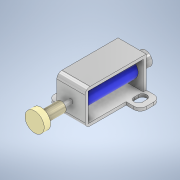
# Autodesk Inventor part: Solenoid
Saved by Autodesk Inventor 2021 (Build 250183000, 183)
## iProperties
Created: 2021-02-15
Part Number: Solenoid
Material: Generic
Document SubType Name: Modeling
Designer: Ryan
Density: 1 g/cm^3
Appearance: Default
Author: Ryan
Autodesk Inventor part; units mm, degrees
ref_plane "YZ Plane" through (0, 0, 0) normal (1, 0, 0) x (0, 1, 0)
ref_plane "XZ Plane" through (0, 0, 0) normal (0, 1, 0) x (-1, 0, 0)
sketch "Sketch1" plane through (0, 0, 0) normal (0, 1, 0) x (-1, 0, 0)
  line L0 (7, 15.2) -> (-7, 15.2)
  line L1 (-7, 15.2) -> (-7, -15.2)
  line L2 (-7, -15.2) -> (7, -15.2)
  line L3 (7, -15.2) -> (7, 15.2)
  point P0 (0, 0)
  dimension "d0" = 30.4
  dimension "d1" = 14
  dimension "d2" = 7
  dimension "d3" = 15.2
  constraints: 8 end point, 2 parallel, 1 horizontal, 1 perpendicular
  measures "d0" distance of L2.end L0.start
  measures "d1" distance of L0.start L0.end
  measures "d2" distance from line of point (0, 0) L3
  measures "d3" distance from line of point (0, 0) L0
extrude "Extrusion1" add sketch "Sketch1" along normal blind 17
fillet "Fillet1" radius 2.54 2 edges at (0, 17, 15.2) (0, 0, 15.2)
sketch "Sketch2" plane through (7, 0, -15.2) normal (1, 0, 0) x (0, 0, -1)
  line L0 (-1.5, 15.5) -> (-28.9, 15.5)
  line L1 (-28.9, 15.5) -> (-28.9, 1.5)
  line L2 (-28.9, 1.5) -> (-1.5, 1.5)
  line L3 (-1.5, 1.5) -> (-1.5, 15.5)
  line L4 (-28.9, 8.5) -> (-30.4, 8.5) construction
  line L5 (-30.4, 2.54) -> (-30.4, 14.46) projected
  line L6 (-1.5, 9.1916) -> (0, 9.1916) construction
  line L7 (0, 0) -> (0, 17) projected
  line L8 (-13.3503, 1.5) -> (-13.3503, 0) construction
  line L9 (-15.2, 15.5) -> (-15.2, 17) construction
  line L10 (0, 17) -> (-27.86, 17) projected
  line L11 (-27.86, 0) -> (0, 0) projected
  point P0 (-15.2, 0)
  dimension "d7" = 1.5
  constraints: 16 end point, 5 point on line, 3 equal length, 3 midpoint, 3 parallel, 2 horizontal, 2 vertical, 1 perpendicular
  measures "d7" distance between parallel lines of L11 L2
extrude "Extrusion2" cut sketch "Sketch2" against normal blind 17
ref_plane "Work Plane1" through (0, 8.5, 0) normal (0, 1, 0) x (1, 0, 0)
sketch "Sketch4" plane through (0, 17, 0) normal (0, 1, 0) x (1, 0, 0)
  line L0 (7, 15.2) -> (-7, 15.2) projected
  line L1 (0, 15.2) -> (3.45, 15.2)
  line L2 (3.45, 15.2) -> (3.45, 21.8)
  line L3 (3.45, 21.8) -> (0, 21.8)
  line L4 (0, 21.8) -> (0, 15.2)
  line L5 (-7, -15.2) -> (7, -15.2) projected
  line L6 (0, 15.2) -> (4.5, 15.2)
  line L7 (4.5, 15.2) -> (4.5, -15.2)
  line L8 (4.5, -15.2) -> (0, -15.2)
  line L9 (0, -15.2) -> (0, 15.2)
  line L10 (1, -15.2) -> (0, -15.2)
  line L11 (0, -15.2) -> (0, -20.1)
  line L12 (0, -20.1) -> (1, -20.1)
  line L13 (1, -20.1) -> (1, -15.2)
  line L14 (0, -20.1) -> (2.5, -20.1)
  line L15 (2.5, -20.1) -> (2.5, -30.1)
  line L16 (2.5, -30.1) -> (0, -30.1)
  line L17 (0, -30.1) -> (0, -20.1)
  point P0 (0, 0)
  dimension "d10" = 3.45
  dimension "d11" = 51.9
  dimension "d12" = 10
  dimension "d14" = 4.9
  dimension "d15" = 2.5
  dimension "d16" = 1
  dimension "d17" = 4.5
  constraints: 32 end point, 8 parallel, 4 horizontal, 4 perpendicular, 3 point on line, 1 midpoint
  measures "d10" distance of L2.end L3.end
  measures "d11" distance between parallel lines of L16 L3
  measures "d12" distance of L14.end L15.end
  measures "d14" distance of L12.end L10.start
  measures "d15" distance of L15.end L16.end
  measures "d16" distance between parallel lines of L11 L13
  measures "d17" distance between parallel lines of L9 L7
sketch "Sketch5" plane through (0, 8.5, 0) normal (0, 1, 0) x (1, 0, 0)
  line L0 (0, 15.2) -> (3.45, 15.2)
  line L1 (3.45, 15.2) -> (3.45, 21.8)
  line L2 (3.45, 21.8) -> (0, 21.8)
  line L3 (0, 21.8) -> (0, 15.2)
  line L4 (0, 15.2) -> (4.5, 15.2)
  line L5 (4.5, 15.2) -> (4.5, -15.2)
  line L6 (4.5, -15.2) -> (0, -15.2)
  line L7 (0, -15.2) -> (0, 15.2)
  line L8 (1, -15.2) -> (0, -15.2)
  line L9 (0, -15.2) -> (0, -20.1)
  line L10 (0, -20.1) -> (1, -20.1)
  line L11 (1, -20.1) -> (1, -15.2)
  line L12 (0, -20.1) -> (2.5, -20.1)
  line L13 (2.5, -20.1) -> (2.5, -30.1)
  line L14 (2.5, -30.1) -> (0, -30.1)
  line L15 (0, -30.1) -> (0, -20.1)
  point P0 (0, 0)
  dimension "d18" = 3.45
  dimension "d19" = 51.9
  dimension "d20" = 10
  dimension "d21" = 4.9
  dimension "d22" = 2.5
  dimension "d23" = 1
  dimension "d24" = 4.5
  constraints: 32 end point, 8 parallel, 4 horizontal, 4 perpendicular, 2 point on line
  measures "d18" distance of L1.end L2.end
  measures "d19" distance between parallel lines of L14 L2
  measures "d20" distance of L12.end L13.end
  measures "d21" distance of L10.end L8.start
  measures "d22" distance of L13.end L14.end
  measures "d23" distance between parallel lines of L9 L11
  measures "d24" distance between parallel lines of L7 L5
revolve "Revolution1" add sketch "Sketch5" angle 360 about axis through (0, 8.5, 30.1) along (0, 0, -1)
sketch "Sketch6" plane through (0, 0, 0) normal (0, 1, 0) x (-1, 0, 0)
  line L0 (-7, -15.2) -> (7, -15.2) projected
  line L1 (-7, 12.66) -> (7, 12.66) projected
  line L2 (7, 12.66) -> (10.825, 12.66)
  line L3 (14, 9.485) -> (14, 5.835)
  line L4 (10.825, 2.66) -> (7, 2.66)
  line L5 (7, 2.66) -> (7, 12.66)
  line L6 (11.25, 6.66) -> (7, 6.66)
  line L7 (7, 6.66) -> (7, 8.66)
  line L8 (7, 8.66) -> (11.25, 8.66)
  line L9 (11.25, 8.66) -> (11.25, 6.66)
  line L10 (7, -15.2) -> (7, 12.66) projected
  line L11 (7, 7.66) -> (14, 7.66) construction
  circle A0 centre (9.125, 6.66) radius 2.125
  circle A1 centre (9.125, 8.66) radius 2.125
  arc A2 (10.825, 2.66) -> (14, 5.835) centre (10.825, 5.835) ccw
  arc A3 (14, 9.485) -> (10.825, 12.66) centre (10.825, 9.485) ccw
  line L12 (-1, 15.2) -> (1, 15.2) projected
  line L13 (7, -15.2) -> (7, 12.66) projected
  line L14 (7, 12.66) -> (7, -15.2)
  line L15 (7, -1.27) -> (-7, -1.27) construction
  line L16 (-7, -13.7) -> (-7, 13.7) projected
  line L17 (0, -1.27) -> (0, -15.2) construction
  line L18 (7, -15.2) -> (10.825, -15.2) construction
  line L19 (14, -12.025) -> (14, -8.375) construction
  line L20 (10.825, -5.2) -> (7, -5.2) construction
  line L21 (7, -5.2) -> (7, -15.2) construction
  line L22 (11.25, -9.2) -> (7, -9.2) construction
  line L23 (7, -9.2) -> (7, -11.2) construction
  line L24 (7, -11.2) -> (11.25, -11.2) construction
  line L25 (11.25, -11.2) -> (11.25, -9.2) construction
  line L26 (7, -10.2) -> (14, -10.2) construction
  circle A4 centre (9.125, -9.2) radius 2.125 construction
  circle A5 centre (9.125, -11.2) radius 2.125 construction
  arc A6 (14, -8.375) -> (10.825, -5.2) centre (10.825, -8.375) ccw construction
  arc A7 (10.825, -15.2) -> (14, -12.025) centre (10.825, -12.025) ccw construction
  line L27 (-7, -5.2) -> (-7, -15.2)
  line L28 (-7, -9.2) -> (-7, -11.2)
  line L29 (-7, -15.2) -> (-10.825, -15.2)
  line L30 (-7, -11.2) -> (-11.25, -11.2)
  line L31 (-11.25, -9.2) -> (-7, -9.2)
  line L32 (-11.25, -11.2) -> (-11.25, -9.2)
  circle A8 centre (-9.125, -11.2) radius 2.125
  circle A9 centre (-9.125, -9.2) radius 2.125
  arc A10 (-14, -12.025) -> (-10.825, -15.2) centre (-10.825, -12.025) ccw
  line L33 (-10.825, -5.2) -> (-7, -5.2)
  line L34 (-7, -10.2) -> (-14, -10.2) construction
  line L35 (-14, -12.025) -> (-14, -8.375)
  arc A11 (-10.825, -5.2) -> (-14, -8.375) centre (-10.825, -8.375) ccw
  point P0 (14, 2.66)
  point P1 (14, 12.66)
  point P2 (14, -5.2)
  point P3 (14, -15.2)
  point P4 (-14, -15.2)
  point P5 (-14, -5.2)
  dimension "d26" = 4.25
  dimension "d27" = 7
  dimension "d28" = 10
  dimension "d29" = 2
  dimension "d30" = 3.175
  constraints: 60 end point, 34 symmetric about line, 14 point on line, 12 point on circle, 7 midpoint, 6 centre point, 5 horizontal, 4 parallel, 4 tangent, 3 perpendicular, 2 horizontal alignment, 2 vertical, 1 collinear, 1 equal radius, 20 other
  measures "d26" distance of L6.start L6.end
  measures "d27" distance of L1.end point (14, 12.66)
  measures "d28" distance of point (14, 12.66) point (14, 2.66)
  measures "d29" distance between parallel lines of L8 L6
  measures "d30" radius of A2
extrude "Extrusion3" add sketch "Sketch6" along normal blind 1.5 contours L29 A10 L35 A11 L33 L16 A9 L32 A8 L27 | L5 A0 L9 A1 L2 A3 L3 A2 L4
sketch "Sketch7" plane through (0, 8.5, 30.1) normal (0, 0, 1) x (1, 0, 0)
  circle A0 centre (0, 0) radius 2.5 projected
  circle A1 centre (0, 0) radius 4.7625
  point P0 (0, -8.5)
  dimension "d33" = 9.525
  constraints: 1 centre point, 1 coincident
  measures "d33" diameter of A1
extrude "Extrusion4" add sketch "Sketch7" along normal blind 3.175 contours A0 | A1
equation "\"d2\" = 0.5 * d1"
equation "\"d3\" = 0.5 * d0"
body "Solid1"
